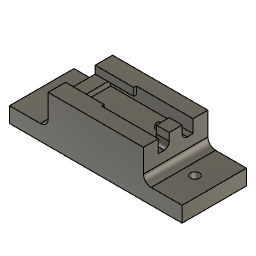
Držák napínacího kolečka v5 (Autodesk Fusion 360 design; units mm, degrees)
Autodesk Fusion 360 part; units mm, degrees
note: some values were not read from the file. Set by a fixed rule: which face or edge a step refers to.
sketch "Sketch1" plane through (0, 0, 0) normal (1, 0, 0) x (0, 1, 0)
  line L0 (0, 0) -> (25, 0)
  line L1 (25, 0) -> (25, 18)
  line L2 (0, 18) -> (0, 0)
  line L3 (19.25, 15) -> (19.25, 13)
  line L4 (19.25, 13) -> (5.75, 13)
  line L5 (5.75, 13) -> (5.75, 15)
  line L6 (18.25, 18) -> (18.25, 15)
  line L7 (6.75, 15) -> (6.75, 18)
  line L8 (25, 18) -> (18.25, 18)
  line L9 (6.75, 18) -> (0, 18)
  line L10 (5.75, 15) -> (6.75, 15)
  line L11 (18.25, 15) -> (19.25, 15)
  line L12 (6.75, 15) -> (18.25, 15)
  line L13 (5.75, 13) -> (19.25, 13)
  line L14 (19.25, 13) -> (19.25, 18)
  line L15 (19.25, 18) -> (5.75, 18)
  line L16 (5.75, 18) -> (5.75, 13)
  dimension "d1" = 25
  dimension "d2" = 18
  dimension "d3" = 13.5
  dimension "d4" = 2
  dimension "d5" = 13
  dimension "d6" = 5.75
  dimension "d7" = 1
  dimension "d8" = 11.5
  dimension "d9" = 3
  dimension "d10" = 15
  dimension "d32" = 13.5
  constraint horizontal L0
  constraint vertical L1
  constraint horizontal L8
  constraint vertical L2
  constraint coincident L0.start L2.end
  constraint horizontal L10
  constraint vertical L3
  constraint horizontal L4
  constraint vertical L5
  constraint vertical L6
  constraint vertical L7
  constraint collinear L8 L9
  constraint collinear L10 L11
  constraint horizontal L13
  constraint vertical L14
  constraint horizontal L15
  constraint vertical L16
  constraint coincident L8 L14.end
  measures "d1" distance of L0.start L0.end
  measures "d2" distance of L0.end L1.end
  measures "d3" distance of L5.end L3.start
  measures "d4" distance of L3.start L3.end
  measures "d5" vertical distance of L0.start L4.end
  measures "d6" horizontal distance of L0.start L4.end
  measures "d7" horizontal distance of L5.end L7.start
  measures "d8" distance of L6.end L7.start
  measures "d9" distance of L7.end L7.start
  measures "d10" vertical distance of L0.start L7.start
  measures "d32" distance of L14.end L15.end
sketch "Bokorys" plane through (0, 0, 0) normal (0, 1, 0) x (1, 0, 0)
  line L0 (-15, 0) -> (52, 0)
  line L1 (52, 0) -> (52, -6)
  line L2 (-15, -6) -> (-15, 0)
  line L3 (-15, -6) -> (52, -6)
  dimension "d48" = 15
  dimension "d49" = 67
  dimension "d50" = 6
  constraint horizontal L0
  constraint vertical L1
  constraint vertical L2
  constraint horizontal L3
  constraint coincident L2.end L0
  constraint coincident L2 L0.start
  measures "d48" distance of origin L0.start
  measures "d49" distance of L0.end L0.start
  measures "d50" distance of L0.end L1.end
extrude "Extrude1" add sketch "Sketch1" along normal blind 15 contours L0 L1 L2 L3 L4 L5 L8 L9 L13 L14 L16 | L7 L9 L10 L15 L16 | L6 L8 L11 L14 L15 makes body 1
extrude "Extrude2" add sketch "Sketch1" along normal blind 5 contours L3 L4 L5 L10 L11 L12 L13 L14 L16 bodies 1
extrude "Extrude3" add sketch "Sketch1" along normal blind 25 contours L0 L1 L2 L3 L4 L5 L8 L9 L13 L14 L16 bodies 1
extrude "Extrude4" add 1 faces at (25, 10.25, 4.3333) along direction (1, 0, 0) blind 2 on bodies 1 bodies 1
sketch "Sketch4" plane through (27, 0, 0) normal (1, 0, 0) x (0, 1, 0)
  line L0 (0, 18) -> (0, 0)
  line L1 (0, 0) -> (25, 0)
  line L2 (25, 0) -> (25, 18)
  line L3 (25, 18) -> (19.25, 18)
  line L4 (19.25, 18) -> (19.25, 13)
  line L5 (19.25, 13) -> (5.75, 13)
  line L6 (5.75, 13) -> (5.75, 18)
  line L7 (5.75, 18) -> (0, 18)
  line L8 (0, 0) -> (25, 0)
  line L9 (25, 0) -> (25, 18)
  line L10 (25, 18) -> (0, 18)
  line L11 (0, 18) -> (0, 0)
  circle A0 centre (12.5, 15.5) radius 1.25
  line L12 (10, 18) -> (15, 18)
  line L13 (15, 18) -> (15, 13)
  line L14 (15, 13) -> (10, 13)
  line L15 (10, 13) -> (10, 18)
  dimension "d39" = 2.5
  dimension "d40" = 2.5
  dimension "d41" = 25
  dimension "d42" = 12.5
  dimension "d57" = 13
  dimension "d59" = 2.5
  dimension "d60" = 5
  dimension "d61" = 5
  constraint horizontal L8
  constraint vertical L9
  constraint horizontal L10
  constraint vertical L11
  constraint coincident L2.end L3.start
  constraint coincident L0.end L1.start
  constraint horizontal L12
  constraint vertical L13
  constraint horizontal L14
  constraint vertical L15
  measures "d39" diameter of A0
  measures "d40" vertical distance of L4.end A0.centre
  measures "d41" distance of L0.end L1.end
  measures "d42" horizontal distance of A0.centre L0.end
  measures "d57" vertical distance of L0.end L14.end
  measures "d59" horizontal distance of A0.centre L14.end
  measures "d60" distance of L12.start L12.end
  measures "d61" distance of L12.end L13.end
extrude "Extrude5" add sketch "Sketch4" along normal blind 5 separate body contours L0 L1 L2 L3 L4 L5 L6 L7 L8 L9 L10 L11 L14 | L5 L6 L10 L15 | L5 L10 L12 L13 L14 L15 | L4 L5 L10 L13 | A0 makes body 2
extrude "Extrude6" add sketch "Sketch4" against normal blind 3 separate body contours A0 makes body 3
extrude "Extrude7" cut 1 faces at (24, 12.8855, 15.0845) along direction (1, 0, 0) blind 1 on bodies 3 bodies 3
extrude "Extrude8" add sketch "Bokorys" along normal blind 25 separate body makes body 4
combine "Combine1" operation add target body 4 tool bodies 2 1
fillet "Fillet1" radius 3 1 edges at (32, 12.5, 6) on bodies 4
fillet "Fillet2" radius 3 1 edges at (0, 12.5, 6) on bodies 4
extrude "Extrude9" add sketch "Sketch4" along normal blind 5 contours L5 L10 L12 L13 L14 L15 | A0 bodies 3
extrude "Extrude10" cut sketch "Sketch4" along normal blind 5 contours L5 L6 L10 L15 | L4 L5 L10 L13 bodies 4
fillet "Fillet3" radius 2 1 edges at (29.5, 10, 13) on bodies 4
fillet "Fillet4" radius 2 1 edges at (29.5, 15, 13) on bodies 4
combine "Combine2" operation add target body 4 tool bodies 3
move_face "OffsetFaces1" offset 5 1 faces at (32, 1.9167, 13.3333) on bodies 4
move_face "OffsetFaces2" offset -5 1 faces at (27, 12.4689, 17.5822) on bodies 4
move_face "OffsetFaces3" offset -5 1 faces at (25, 12.8855, 15.0845) on bodies 4
sketch "Sketch6" plane through (0, 0, 6) normal (0, 0, 1) x (-1, 0, 0)
  line L0 (3, 0) -> (3, -25)
  line L1 (3, -25) -> (15, -25)
  line L2 (15, -25) -> (15, 0)
  line L3 (15, 0) -> (3, 0)
  line L4 (15, -25) -> (-52, -25)
  line L5 (-52, -25) -> (-52, 0)
  line L6 (-52, 0) -> (15, 0)
  line L7 (15, 0) -> (15, -25)
  circle A0 centre (7.5, -12.5) radius 1.75
  line L8 (-18.5, -37) -> (-18.5, 8) construction
  circle A1 centre (-44.5, -12.5) radius 1.75
  dimension "d73" = 3.5
  dimension "d74" = 12.5
  dimension "d75" = 7.5
  dimension "d76" = 33.5
  dimension "d77" = 67
  constraint horizontal L4
  constraint vertical L5
  constraint horizontal L6
  constraint vertical L7
  constraint coincident L1.end L2.start
  constraint vertical L8
  constraint symmetric A0 L8 A1
  measures "d73" diameter of A0
  measures "d74" vertical distance of origin A0.centre
  measures "d75" horizontal distance of L2.end A0.centre
  measures "d76" distance of L2.end L8
  measures "d77" distance of L1.end L4.end
extrude "Extrude13" cut sketch "Sketch6" against normal blind 16 contours A0 | A1 bodies 4
extrude "Extrude11" [suppressed]
extrude "Extrude12" [suppressed]
